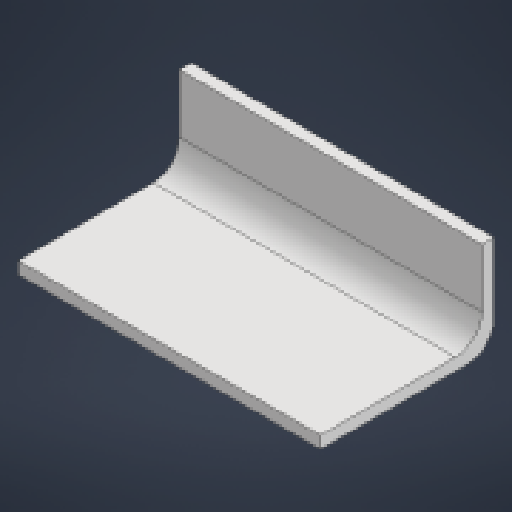
# Autodesk Inventor part: 前舵机位置控制
Saved by Autodesk Inventor 2025 (Build 290162000, 162)
## iProperties
Created: 2025-12-02
Part Number: 前舵机位置控制
Material: 常规
Document SubType Name: Modeling
Designer: HZD
Density: 1 g/cm^3
Appearance: 默认
Author: HZD
Autodesk Inventor part; units mm, degrees
ref_plane "YZ Plane" through (0, 0, 0) normal (1, 0, 0) x (0, 1, 0)
ref_plane "XZ Plane" through (0, 0, 0) normal (0, 1, 0) x (-1, 0, 0)
ref_plane "XY Plane" through (0, 0, 0) normal (0, 0, 1) x (1, 0, 0)
sketch "草图2" plane through (0, 0, 0) normal (0, 1, 0) x (-1, 0, 0)
  line L0 (-70.613, -25.5176) -> (4.387, -25.5176) projected
  line L1 (-70.613, -25.5176) -> (-70.613, 14.4824) projected
  line L2 (4.387, 14.4824) -> (-70.613, 14.4824) projected
  line L3 (4.387, -25.5176) -> (4.387, 14.4824) projected
  point P0 (0, 0)
extrude "拉伸1" add sketch "草图2" along normal blind 3
sketch "草图3" plane through (-4.387, 0, -25.5176) normal (-1, 0, 0) x (0, 0, 1)
  line L0 (0, 0) -> (40, 0) projected
  line L1 (0, 0) -> (-3, 0)
  line L2 (-3, 0) -> (-3, 26)
  line L3 (-3, 26) -> (0, 26)
  line L4 (0, 26) -> (0, 0)
  point P0 (25.5176, 0)
  dimension "d2" = 3
  dimension "d3" = 26
  constraints: 8 end point, 2 parallel, 1 horizontal, 1 perpendicular
  measures "d2" distance of L2.end L3.end
  measures "d3" distance between parallel lines of L1 L3
extrude "拉伸2" add sketch "草图3" against normal up to surface (75 mm away)
fillet "圆角1" radius 6.5 2 edges at (33.113, 3, -25.5176) (33.113, 0, -28.5176)
sketch "草图4" plane through (70.613, 26, -28.5176) normal (0, 0, -1) x (-1, 0, 0)
  line L0 (0, -1.1) -> (75, -1.1) projected
  line L1 (0, -76.1) -> (0, -1.1) projected
  line L2 (75, -76.1) -> (0, -76.1) projected
  line L3 (75, -1.1) -> (75, -76.1) projected
  line L4 (78, -79.1) -> (-3, -79.1)
  line L5 (-3, -79.1) -> (-3, 1.9)
  line L6 (-3, 1.9) -> (78, 1.9)
  line L7 (78, 1.9) -> (78, -79.1)
  line L8 (78, -8.1) -> (-3, -8.1)
  line L9 (68, 1.9) -> (68, -79.1)
  line L10 (37.5, -29.6254) -> (37.5, -58.9595)
  line L11 (7, 1.9) -> (7, -79.1)
  point P0 (70.613, -26)
  point P1 (0, -8.1)
  point P2 (75, -8.1)
  dimension "d8" = 3
  dimension "d9" = 10
  dimension "d10" = 10
  constraints: 16 end point, 4 point on line, 2 perpendicular, 2 symmetric about line, 1 vertical, 3 other
  measures "d8" distance between parallel lines of L3 L7
  measures "d9" distance between parallel lines of L6 L8
  measures "d10" distance between parallel lines of L7 L9
extrude "拉伸3" add sketch "草图4" along normal blind 2 contours L1 L8 L5 L6 L11 L0 | L11 L6 L9 L0 | L9 L6 L7 L8 L3 L0
sketch "草图5" plane through (70.613, 26, -28.5176) normal (0, 0, 1) x (1, 0, 0)
  line L0 (0, 0) -> (0, -1.1) projected
  line L1 (0, -1.1) -> (0, -8.1) projected
  line L2 (3, -8.1) -> (0, -8.1) projected
  line L3 (3, 1.9) -> (3, -8.1) projected
  line L4 (-78, 1.9) -> (3, 1.9) projected
  line L5 (-78, -8.1) -> (-78, 1.9) projected
  line L6 (-75, -8.1) -> (-78, -8.1) projected
  line L7 (-75, -1.1) -> (-75, -8.1) projected
  line L8 (-75, 0) -> (-75, -1.1) projected
  line L9 (-75, 0) -> (0, 0) projected
  point P0 (-70.613, -26)
extrude "拉伸4" add sketch "草图5" along normal up to surface (3 mm away)
fillet "圆角2" radius 3 2 edges at (-4.387, 17.9, -27.0176) (70.613, 17.9, -27.0176)
